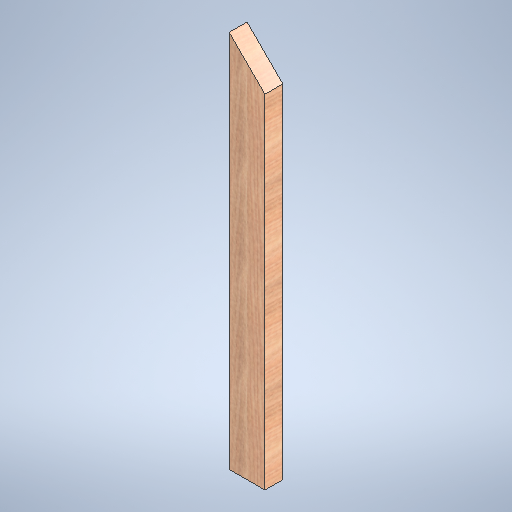
# Autodesk Inventor part: 2x4x42.343 (45 90)
Saved by Autodesk Inventor 2025 (Build 290162000, 162)
## iProperties
Created: 2024-07-01
Part Number: 2x4x42.343 (45 90)
Material: Generic
Document SubType Name: Modeling
Designer: Cupri
Density: 1 g/cm^3
Appearance: Default
Author: Cupri
Autodesk Inventor part; units mm, degrees
ref_plane "YZ Plane" through (0, 0, 0) normal (1, 0, 0) x (0, 1, 0)
ref_plane "XZ Plane" through (0, 0, 0) normal (0, 1, 0) x (-1, 0, 0)
ref_plane "XY Plane" through (0, 0, 0) normal (0, 0, 1) x (1, 0, 0)
sketch "Sketch1" plane through (0, 0, 0) normal (0, 0, 1) x (1, 0, 0)
  line L0 (0, 0) -> (0, 1075.5122)
  line L1 (0, 0) -> (101.6, 0)
  line L2 (101.6, 0) -> (101.6, 973.9122)
  line L3 (101.6, 973.9122) -> (0, 1075.5122)
  dimension "d0" = 1075.5122
  dimension "d1" = 101.6
  dimension "d2" = 973.9122
  constraints: 8 end point, 2 vertical, 1 horizontal
  measures "d0" distance of L0.start L0.end
  measures "d1" distance of L0.start L1.end
  measures "d2" distance of L1.end L2.end
extrude "Extrusion1" add sketch "Sketch1" along normal blind 50.8
body "Solid1"
